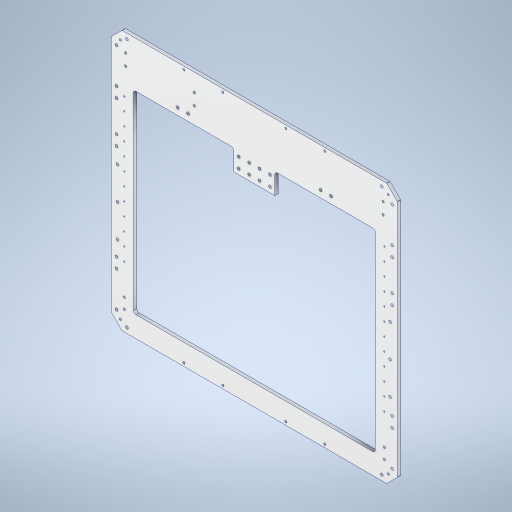
# Autodesk Inventor part: Printer Gantry Plate RevII
Saved by Autodesk Inventor 2024 (Build 280153000, 153)
## iProperties
Created: 2024-10-26
Part Number: Printer Gantry Plate RevII
Material: Aluminum 6061
Document SubType Name: Modeling
Designer: Ishaan
Density: 2.7 g/cm^3
Appearance: Aluminum - Flat
Author: Ishaan
Autodesk Inventor part; units mm, degrees
ref_plane "YZ Plane" through (0, 0, 0) normal (1, 0, 0) x (0, 1, 0)
ref_plane "XZ Plane" through (0, 0, 0) normal (0, 1, 0) x (-1, 0, 0)
ref_plane "XY Plane" through (0, 0, 0) normal (0, 0, 1) x (1, 0, 0)
sketch "Sketch1" plane through (0, 0, 0) normal (0, 0, 1) x (1, 0, 0)
  line L0 (275, -250) -> (-275, -250)
  line L1 (-275, -250) -> (-275, 250)
  line L2 (-275, 250) -> (275, 250)
  line L3 (275, 250) -> (275, -250)
  line L4 (275, -250) -> (-275, 250) construction
  line L5 (-275, -250) -> (275, 250) construction
  point P0 (0, 0)
  dimension "d0" = 550
  dimension "d1" = 500
  constraints: 12 end point, 2 midpoint, 2 parallel, 1 horizontal, 1 perpendicular
  measures "d0" distance of L1.end L2.end
  measures "d1" distance of L0.end L1.end
extrude "Extrusion1" add sketch "Sketch1" against normal blind 6.35
sketch "Sketch2" plane through (0, 0, 0) normal (0, 0, 1) x (1, 0, 0)
  line L0 (-235, 210) -> (-275, 210) construction
  line L1 (-275, 210) -> (-275, 250) construction
  line L2 (-275, 250) -> (-235, 250) construction
  line L3 (-235, 250) -> (-235, 210) construction
  line L4 (-235, 210) -> (-275, 250) construction
  line L5 (-275, 210) -> (-235, 250) construction
  line L6 (275, 210) -> (235, 210) construction
  line L7 (235, 210) -> (235, 250) construction
  line L8 (235, 250) -> (275, 250) construction
  line L9 (275, 250) -> (275, 210) construction
  line L10 (275, 210) -> (235, 250) construction
  line L11 (235, 210) -> (275, 250) construction
  line L12 (40, 122) -> (-40, 122) construction
  line L13 (-40, 122) -> (-40, 162) construction
  line L14 (-40, 162) -> (40, 162) construction
  line L15 (40, 162) -> (40, 122) construction
  line L16 (40, 122) -> (-40, 162) construction
  line L17 (-40, 122) -> (40, 162) construction
  line L18 (-235, -250) -> (-275, -250) construction
  line L19 (-275, -250) -> (-275, -210) construction
  line L20 (-275, -210) -> (-235, -210) construction
  line L21 (-235, -210) -> (-235, -250) construction
  line L22 (-235, -250) -> (-275, -210) construction
  line L23 (-275, -250) -> (-235, -210) construction
  line L24 (-275, 250) -> (-275, -250) construction
  line L25 (-275, -250) -> (275, -250) construction
  line L26 (275, -250) -> (235, -250) construction
  line L27 (235, -250) -> (235, -210) construction
  line L28 (235, -210) -> (275, -210) construction
  line L29 (275, -210) -> (275, -250) construction
  line L30 (275, -250) -> (235, -210) construction
  line L31 (235, -250) -> (275, -210) construction
  line L32 (275, -250) -> (275, 250) construction
  line L33 (-255, 122) -> (-275, 122) construction
  line L34 (-275, 122) -> (-275, 162) construction
  line L35 (-275, 162) -> (-255, 162) construction
  line L36 (-255, 162) -> (-255, 122) construction
  line L37 (-255, 122) -> (-275, 162) construction
  line L38 (-275, 122) -> (-255, 162) construction
  line L39 (275, 122) -> (255, 122) construction
  line L40 (255, 122) -> (255, 162) construction
  line L41 (255, 162) -> (275, 162) construction
  line L42 (275, 162) -> (275, 122) construction
  line L43 (275, 122) -> (255, 162) construction
  line L44 (255, 122) -> (275, 162) construction
  line L45 (-117.5, 165) -> (-157.5, 165) construction
  line L46 (-157.5, 165) -> (-157.5, 185) construction
  line L47 (-157.5, 185) -> (-117.5, 185) construction
  line L48 (-117.5, 185) -> (-117.5, 165) construction
  line L49 (-117.5, 165) -> (-157.5, 185) construction
  line L50 (-157.5, 165) -> (-117.5, 185) construction
  line L51 (157.5, 165) -> (117.5, 165) construction
  line L52 (117.5, 165) -> (117.5, 185) construction
  line L53 (117.5, 185) -> (157.5, 185) construction
  line L54 (157.5, 185) -> (157.5, 165) construction
  line L55 (157.5, 165) -> (117.5, 185) construction
  line L56 (117.5, 165) -> (157.5, 185) construction
  line L57 (-137.5, 175) -> (137.5, 175) construction
  line L58 (-255, -162) -> (-275, -162) construction
  line L59 (-275, -162) -> (-275, -122) construction
  line L60 (-275, -122) -> (-255, -122) construction
  line L61 (-255, -122) -> (-255, -162) construction
  line L62 (-255, -162) -> (-275, -122) construction
  line L63 (-275, -162) -> (-255, -122) construction
  line L64 (-255, 42) -> (-275, 42) construction
  line L65 (-275, 42) -> (-275, 82) construction
  line L66 (-275, 82) -> (-255, 82) construction
  line L67 (-255, 82) -> (-255, 42) construction
  line L68 (-255, 42) -> (-275, 82) construction
  line L69 (-275, 42) -> (-255, 82) construction
  line L70 (275, 42) -> (255, 42) construction
  line L71 (255, 42) -> (255, 82) construction
  line L72 (255, 82) -> (275, 82) construction
  line L73 (275, 82) -> (275, 42) construction
  line L74 (275, 42) -> (255, 82) construction
  line L75 (255, 42) -> (275, 82) construction
  line L76 (275, -162) -> (255, -162) construction
  line L77 (255, -162) -> (255, -122) construction
  line L78 (255, -122) -> (275, -122) construction
  line L79 (275, -122) -> (275, -162) construction
  line L80 (275, -162) -> (255, -122) construction
  line L81 (255, -162) -> (275, -122) construction
  line L82 (-275, 220) -> (-235, 220) construction
  line L83 (-275, -250) -> (-275, 250) construction
  line L84 (-275, 132) -> (-255, 132) construction
  line L85 (-275, -220) -> (-235, -220) construction
  line L86 (-275, -132) -> (-255, -132) construction
  line L87 (-255, 42) -> (-255, -122) construction
  line L88 (-255, -40) -> (0, -40) construction
  line L89 (0, 122) -> (0, -250) construction
  line L90 (-245, 220) -> (-265, 220) construction
  line L91 (-265, 220) -> (-265, 240) construction
  line L92 (-265, 240) -> (-245, 240) construction
  line L93 (-245, 240) -> (-245, 220) construction
  line L94 (-245, 220) -> (-265, 240) construction
  line L95 (-265, 220) -> (-245, 240) construction
  line L96 (265, 220) -> (245, 220) construction
  line L97 (245, 220) -> (245, 240) construction
  line L98 (245, 240) -> (265, 240) construction
  line L99 (265, 240) -> (265, 220) construction
  line L100 (265, 220) -> (245, 240) construction
  line L101 (245, 220) -> (265, 240) construction
  line L102 (265, 152) -> (265, 132) construction
  line L103 (265, 72) -> (265, 52) construction
  line L104 (265, -132) -> (265, -152) construction
  line L105 (-265, 152) -> (-265, 132) construction
  line L106 (-265, 72) -> (-265, 52) construction
  line L107 (-265, -132) -> (-265, -152) construction
  line L108 (-147.5, 175) -> (-127.5, 175) construction
  line L109 (127.5, 175) -> (147.5, 175) construction
  line L110 (265, -240) -> (245, -240) construction
  line L111 (245, -240) -> (245, -220) construction
  line L112 (245, -220) -> (265, -220) construction
  line L113 (265, -220) -> (265, -240) construction
  line L114 (265, -240) -> (245, -220) construction
  line L115 (245, -240) -> (265, -220) construction
  line L116 (-245, -240) -> (-265, -240) construction
  line L117 (-265, -240) -> (-265, -220) construction
  line L118 (-265, -220) -> (-245, -220) construction
  line L119 (-245, -220) -> (-245, -240) construction
  line L120 (-245, -240) -> (-265, -220) construction
  line L121 (-265, -240) -> (-245, -220) construction
  line L122 (10, 132) -> (-10, 132) construction
  line L123 (-10, 132) -> (-10, 152) construction
  line L124 (-10, 152) -> (10, 152) construction
  line L125 (10, 152) -> (10, 132) construction
  line L126 (10, 132) -> (-10, 152) construction
  line L127 (-10, 132) -> (10, 152) construction
  line L128 (30, 132) -> (-30, 132) construction
  line L129 (-30, 132) -> (-30, 152) construction
  line L130 (-30, 152) -> (30, 152) construction
  line L131 (30, 152) -> (30, 132) construction
  line L132 (30, 132) -> (-30, 152) construction
  line L133 (-30, 132) -> (30, 152) construction
  point P0 (0, 0)
  point P1 (-255, 230)
  point P2 (255, 230)
  point P3 (0, 142)
  point P4 (-255, -230)
  point P5 (255, -230)
  point P6 (0, 175)
  point P7 (265, 142)
  point P8 (265, 62)
  point P9 (265, -142)
  point P10 (-265, -142)
  point P11 (-265, 62)
  point P12 (-265, 142)
  point P13 (0, 142)
  dimension "d4" = 40
  dimension "d5" = 40
  dimension "d6" = 40
  dimension "d7" = 40
  dimension "d8" = 80
  dimension "d9" = 40
  dimension "d10" = 40
  dimension "d11" = 40
  dimension "d13" = 40
  dimension "d14" = 40
  dimension "d15" = 20
  dimension "d16" = 40
  dimension "d17" = 20
  dimension "d18" = 40
  dimension "d19" = 40
  dimension "d20" = 20
  dimension "d21" = 40
  dimension "d22" = 20
  dimension "d23" = 3
  dimension "d24" = 275
  dimension "d25" = 20
  dimension "d26" = 40
  dimension "d27" = 20
  dimension "d28" = 40
  dimension "d29" = 20
  dimension "d30" = 40
  dimension "d31" = 20
  dimension "d32" = 40
  dimension "d33" = 392
  dimension "d35" = 10
  dimension "d36" = 10
  dimension "d37" = 88
  dimension "d40" = 88
  dimension "d42" = 48
  dimension "d44" = 164
  dimension "d49" = 10
  dimension "d51" = 162
  dimension "d52" = 20
  dimension "d53" = 20
  dimension "d54" = 20
  dimension "d55" = 20
  dimension "d56" = 20
  dimension "d57" = 20
  dimension "d58" = 20
  dimension "d59" = 20
  dimension "d60" = 20
  dimension "d61" = 20
  dimension "d62" = 20
  dimension "d63" = 20
  dimension "d64" = 20
  dimension "d65" = 20
  dimension "d66" = 20
  dimension "d67" = 20
  dimension "d68" = 20
  dimension "d69" = 20
  dimension "d70" = 60
  dimension "d71" = 20
  dimension "d79" = 10
  dimension "d87" = 80
  constraints: 260 end point, 52 midpoint, 38 parallel, 33 coincident, 23 perpendicular, 22 horizontal, 13 collinear, 6 vertical, 5 point on line, 2 horizontal alignment, 2 vertical alignment, 4 other
  measures "d4" distance of L1.end L2.end
  measures "d5" distance of L0.end L1.end
  measures "d6" distance of L7.end L8.end
  measures "d7" distance of L6.end L7.end
  measures "d8" distance of L13.end L14.end
  measures "d9" distance of L12.end L13.end
  measures "d10" distance of L19.end L20.end
  measures "d11" distance of L18.end L19.end
  measures "d13" distance of L27.end L28.end
  measures "d14" distance of L26.end L27.end
  measures "d15" distance of L34.end L35.end
  measures "d16" distance of L33.end L34.end
  measures "d17" distance of L40.end L41.end
  measures "d18" distance of L39.end L40.end
  measures "d19" distance of L46.end L47.end
  measures "d20" distance of L45.end L46.end
  measures "d21" distance of L52.end L53.end
  measures "d22" distance of L51.end L52.end
  measures "d23" distance between parallel lines of L14 L45
  measures "d24" distance of L57.start L57.end
  measures "d25" distance of L59.end L60.end
  measures "d26" distance of L58.end L59.end
  measures "d27" distance of L65.end L66.end
  measures "d28" distance of L64.end L65.end
  measures "d29" distance of L71.end L72.end
  measures "d30" distance of L70.end L71.end
  measures "d31" distance of L77.end L78.end
  measures "d32" distance of L76.end L77.end
  measures "d33" distance from line of L25 point (0, 142)
  measures "d35" distance between parallel lines of L82 L0
  measures "d36" distance between parallel lines of L33 L84
  measures "d37" distance between parallel lines of L82 L84
  measures "d40" distance between parallel lines of L86 L85
  measures "d42" distance between parallel lines of L20 L58
  measures "d44" distance between parallel lines of L60 L64
  measures "d49" distance between parallel lines of L60 L86
  measures "d51" distance between parallel lines of L12 L88
  measures "d52" distance of L91.end L92.end
  measures "d53" distance of L90.end L91.end
  measures "d54" distance of L97.end L98.end
  measures "d55" distance of L96.end L97.end
  measures "d56" distance of L102.start L102.end
  measures "d57" distance of L103.start L103.end
  measures "d58" distance of L104.start L104.end
  measures "d59" distance of L105.start L105.end
  measures "d60" distance of L106.start L106.end
  measures "d61" distance of L107.start L107.end
  measures "d62" distance of L108.start L108.end
  measures "d63" distance of L109.start L109.end
  measures "d64" distance of L111.end L112.end
  measures "d65" distance of L110.end L111.end
  measures "d66" distance of L117.end L118.end
  measures "d67" distance of L116.end L117.end
  measures "d68" distance of L123.end L124.end
  measures "d69" distance of L122.end L123.end
  measures "d70" distance of L129.end L130.end
  measures "d71" distance of L128.end L129.end
  measures "d79" distance between parallel lines of L20 L85
  measures "d87" distance between parallel lines of L66 L35
hole "Hole1" at (-245, 240, 0) at (-265, 220, 0) at (245, 240, 0) at (265, 220, 0) at (265, 152, 0) at (265, 132, 0) at (265, 52, 0) at (265, 72, 0) at (265, -152, 0) at (265, -132, 0) at (-265, 132, 0) at (-265, 152, 0) at (-265, 52, 0) at (-265, 72, 0) at (-265, -152, 0) at (-265, -132, 0) at (-127.5, 175, 0) at (-147.5, 175, 0) at (147.5, 175, 0) at (127.5, 175, 0) at (-265, -220, 0) at (-245, -240, 0) at (245, -240, 0) at (265, -220, 0) at (-30, 152, 0) at (-30, 132, 0) at (-10, 132, 0) at (-10, 152, 0) at (10, 152, 0) at (10, 132, 0) at (30, 132, 0) at (30, 152, 0) direction (0, 0, -1) diameter 5.3 end through all
sketch "Sketch9" plane through (0, 0, 0) normal (0, 0, 1) x (1, 0, 0)
  line L0 (232.5, -210) -> (-232.5, -210)
  line L1 (-232.5, -210) -> (-232.5, 162)
  line L2 (-232.5, 162) -> (232.5, 162)
  line L3 (232.5, 162) -> (232.5, -210)
  line L4 (232.5, -210) -> (-232.5, 162) construction
  line L5 (-232.5, -210) -> (232.5, 162) construction
  line L6 (-275, -250) -> (275, -250) projected
  circle A0 centre (30, 152) radius 2.65 construction
  circle A1 centre (30, 132) radius 2.65 construction
  circle A2 centre (10, 132) radius 2.65 construction
  circle A3 centre (10, 152) radius 2.65 construction
  circle A4 centre (-10, 152) radius 2.65 construction
  circle A5 centre (-10, 132) radius 2.65 construction
  circle A6 centre (-30, 132) radius 2.65 construction
  circle A7 centre (-30, 152) radius 2.65 construction
  circle A8 centre (265, -220) radius 2.65 construction
  circle A9 centre (245, -240) radius 2.65 construction
  circle A10 centre (-245, -240) radius 2.65 construction
  circle A11 centre (-265, -220) radius 2.65 construction
  circle A12 centre (127.5, 175) radius 2.65 construction
  circle A13 centre (147.5, 175) radius 2.65 construction
  circle A14 centre (-147.5, 175) radius 2.65 construction
  circle A15 centre (-127.5, 175) radius 2.65 construction
  circle A16 centre (-265, -132) radius 2.65 construction
  circle A17 centre (-265, -152) radius 2.65 construction
  circle A18 centre (-265, 72) radius 2.65 construction
  circle A19 centre (-265, 52) radius 2.65 construction
  circle A20 centre (-265, 152) radius 2.65 construction
  circle A21 centre (-265, 132) radius 2.65 construction
  circle A22 centre (265, -132) radius 2.65 construction
  circle A23 centre (265, -152) radius 2.65 construction
  circle A24 centre (265, 72) radius 2.65 construction
  circle A25 centre (265, 52) radius 2.65 construction
  circle A26 centre (265, 132) radius 2.65 construction
  circle A27 centre (265, 152) radius 2.65 construction
  circle A28 centre (265, 220) radius 2.65 construction
  circle A29 centre (245, 240) radius 2.65 construction
  circle A30 centre (-265, 220) radius 2.65 construction
  circle A31 centre (-245, 240) radius 2.65 construction
  line L7 (275, 250) -> (-275, 250) construction
  line L8 (-275, 250) -> (-275, -250) construction
  line L9 (-275, -250) -> (275, -250) construction
  line L10 (275, -250) -> (275, 250) construction
  line L11 (-30, 152) -> (30, 132) construction
  line L12 (39.6, 122) -> (-39.6, 122)
  line L13 (-39.6, 122) -> (-39.6, 162)
  line L14 (-39.6, 162) -> (39.6, 162)
  line L15 (39.6, 162) -> (39.6, 122)
  line L16 (39.6, 122) -> (-39.6, 162) construction
  line L17 (-39.6, 122) -> (39.6, 162) construction
  point P0 (0, 0)
  point P1 (0, -24)
  point P2 (0, 142)
  dimension "d148" = 465
  dimension "d150" = 40
  dimension "d151" = 79.2
  dimension "d152" = 40
  dimension "d153" = 13
  constraints: 26 end point, 5 midpoint, 4 parallel, 2 horizontal, 2 perpendicular, 1 vertical alignment
  measures "d148" distance of L1.end L2.end
  measures "d150" distance between parallel lines of L0 L6
  measures "d151" distance of L13.end L14.end
  measures "d152" distance of L12.end L13.end
  measures "d153" distance from line of L2 A13.centre
extrude "Extrusion4" cut sketch "Sketch9" against normal through all contours L0 L1 L2 L13 L12 L15 L3
sketch "Sketch10" plane through (0, 0, 0) normal (0, 0, 1) x (1, 0, 0)
  line L0 (275, 250) -> (-275, 250) projected
  line L1 (-275, 250) -> (-255, 250)
  line L2 (-255, 250) -> (-255, 230)
  line L3 (-255, 230) -> (-275, 230)
  line L4 (-275, 230) -> (-275, 250)
  line L5 (275, 250) -> (275, -250) projected
  line L6 (275, 250) -> (255, 250)
  line L7 (255, 250) -> (255, 230)
  line L8 (255, 230) -> (275, 230)
  line L9 (275, 230) -> (275, 250)
  line L10 (275, -250) -> (255, -250)
  line L11 (255, -250) -> (255, -230)
  line L12 (255, -230) -> (275, -230)
  line L13 (275, -230) -> (275, -250)
  line L14 (-275, -250) -> (-255, -250)
  line L15 (-255, -250) -> (-255, -230)
  line L16 (-255, -230) -> (-275, -230)
  line L17 (-275, -230) -> (-275, -250)
  point P0 (0, 0)
  point P1 (275, -230)
  point P2 (-255, 250)
  dimension "d156" = 20
  dimension "d157" = 20
  constraints: 32 end point, 8 parallel, 4 horizontal, 4 perpendicular, 3 collinear, 3 equal length, 1 point on line
  measures "d156" distance of L2.end L3.end
  measures "d157" distance of L1.end L2.end
extrude "Extrusion5" cut sketch "Sketch10" against normal through all
sketch "Sketch11" plane through (0, 0, 0) normal (0, 0, 1) x (1, 0, 0)
  line L0 (261, -102.5) -> (-263, -102.5) construction
  line L1 (-263, -102.5) -> (-263, 22.5) construction
  line L2 (-263, 22.5) -> (261, 22.5) construction
  line L3 (261, 22.5) -> (261, -102.5) construction
  line L4 (261, -102.5) -> (-263, 22.5) construction
  line L5 (-263, -102.5) -> (261, 22.5) construction
  circle A0 centre (-265, 52) radius 2.65 construction
  circle A1 centre (265, 52) radius 2.65 construction
  circle A2 centre (-265, -132) radius 2.65 construction
  line L6 (-265, 52) -> (-265, -132) construction
  point P0 (0, 0)
  point P1 (-1, -40)
  point P2 (-265, -40)
  point P3 (-263, -40)
  point P4 (261, -40)
  dimension "d160" = 125
  dimension "d161" = 2
  dimension "d162" = 4
  constraints: 14 end point, 5 midpoint, 4 coincident, 2 parallel, 1 horizontal, 1 horizontal alignment, 1 perpendicular, 1 vertical
  measures "d160" distance of L0.end L1.end
  measures "d161" distance from line of L1 L6.start
  measures "d162" distance from line of A1.centre L3
hole "Hole6" at (-263, 22.5, 0) at (-263, -40, 0) at (-263, -102.5, 0) at (261, 22.5, 0) at (261, -40, 0) at (261, -102.5, 0) direction (0, 0, -1) diameter 5.3 end through all
sketch "Sketch12" plane through (0, 0, 0) normal (0, 0, 1) x (1, 0, 0)
  line L0 (-244, -145) -> (-256, -145) construction
  line L1 (-256, -145) -> (-256, 155) construction
  line L2 (-256, 155) -> (-244, 155) construction
  line L3 (-244, 155) -> (-244, -145) construction
  line L4 (-244, -145) -> (-256, 155) construction
  line L5 (-256, -145) -> (-244, 155) construction
  line L6 (-250, 142.5) -> (-250, -132.5) construction
  line L7 (-275, 230) -> (-275, -230) construction
  line L8 (255, 250) -> (-255, 250) construction
  point P0 (0, 0)
  point P1 (-250, 5)
  point P2 (-250, -107.5)
  point P3 (-250, -82.5)
  point P4 (-250, -57.5)
  point P5 (-250, -32.5)
  point P6 (-250, -7.5)
  point P7 (-250, 17.5)
  point P8 (-250, 42.5)
  point P9 (-250, 67.5)
  point P10 (-250, 92.5)
  point P11 (-250, 117.5)
  point P12 (-250, 142.5)
  dimension "d170" = 12
  dimension "d171" = 300
  dimension "d172" = 275
  dimension "d175" = 25
  dimension "d180" = 25
  dimension "d181" = 95
  constraints: 14 end point, 3 midpoint, 2 parallel, 2 vertical, 1 coincident, 1 horizontal, 1 perpendicular, 11 other
  measures "d170" distance of L1.end L2.end
  measures "d171" distance of L0.end L1.end
  measures "d172" distance of L6.start L6.end
  measures "d175" distance of point (-250, -132.5) point (-250, -107.5)
  measures "d180" distance from line of point (-250, 5) L7
  measures "d181" distance between parallel lines of L8 L2
hole "Hole7" at (-250, -132.5, 0) at (-250, -107.5, 0) at (-250, -82.5, 0) at (-250, -57.5, 0) at (-250, -32.5, 0) at (-250, -7.5, 0) at (-250, 17.5, 0) at (-250, 42.5, 0) at (-250, 67.5, 0) at (-250, 92.5, 0) at (-250, 117.5, 0) at (-250, 142.5, 0) direction (0, 0, -1) diameter 2.459 end through all thread size "M3x0.5" class "6H" standard "ANSI Metric M Profile"
mirror "Mirror1" about plane through (0, 0, 0) normal (1, 0, 0) of "Hole7"
sketch "Sketch13" plane through (0, 0, 0) normal (0, 0, 1) x (1, 0, 0)
  line L0 (247.5, 194) -> (-247.5, 194) construction
  line L1 (-247.5, 194) -> (-247.5, 216) construction
  line L2 (-247.5, 216) -> (247.5, 216) construction
  line L3 (247.5, 216) -> (247.5, 194) construction
  line L4 (247.5, 194) -> (-247.5, 216) construction
  line L5 (-247.5, 194) -> (247.5, 216) construction
  line L6 (-115.5, 194) -> (-115.5, 216) construction
  line L7 (255, 250) -> (-255, 250) construction
  line L8 (-275, 230) -> (-275, -230) construction
  line L9 (250, -212) -> (-250, -212) construction
  line L10 (-250, -212) -> (-250, -192) construction
  line L11 (-250, -192) -> (250, -192) construction
  line L12 (250, -192) -> (250, -212) construction
  line L13 (250, -212) -> (-250, -192) construction
  line L14 (-250, -212) -> (250, -192) construction
  line L15 (-255, -250) -> (255, -250) construction
  point P0 (0, 0)
  point P1 (0, 205)
  point P2 (0, -202)
  dimension "d189" = 22
  dimension "d190" = 34
  dimension "d191" = 27.5
  dimension "d192" = 132
  dimension "d193" = 20
  dimension "d194" = 25
  dimension "d195" = 38
  constraints: 26 end point, 10 coincident, 4 midpoint, 4 parallel, 3 perpendicular, 2 horizontal, 2 point on line, 2 vertical alignment
  measures "d189" distance of L0.end L1.end
  measures "d190" distance between parallel lines of L7 L2
  measures "d191" distance between parallel lines of L8 L1
  measures "d192" distance between parallel lines of L6 L1
  measures "d193" distance of L9.end L10.end
  measures "d194" distance between parallel lines of L10 L8
  measures "d195" distance between parallel lines of L15 L9
hole "Hole8" at (-115.5, 216, 0) at (-115.5, 194, 0) at (-247.5, 216, 0) at (-247.5, 194, 0) at (247.5, 216, 0) at (247.5, 194, 0) at (-250, -192, 0) at (-250, -212, 0) at (250, -192, 0) at (250, -212, 0) direction (0, 0, -1) diameter 4.134 end through all thread size "M5x0.8" class "6H" standard "ANSI Metric M Profile"
fillet "Fillet2" radius 5 4 edges at (-232.5, 162, -3.175) (232.5, 162, -3.175) (232.5, -210, -3.175) (-232.5, -210, -3.175)
fillet "Fillet3" radius 5 2 edges at (-39.6, 162, -3.175) (39.6, 162, -3.175)
fillet "Fillet4" radius 1 12 edges at (255, -250, -3.175) (255, -230, -3.175) (275, -230, -3.175) (255, 230, -3.175) (275, 230, -3.175) (255, 250, -3.175) (-255, -230, -3.175) (-275, 230, -3.175) (-255, 230, -3.175) (-255, 250, -3.175) (-255, -250, -3.175) (-275, -230, -3.175)
sketch "Sketch14" plane through (0, 0, 0) normal (0, 0, 1) x (1, 0, 0)
  circle A0 centre (250, -212) radius 2.067 projected
  circle A1 centre (250, -192) radius 2.067 projected
  circle A2 centre (-250, -212) radius 2.067 projected
  circle A3 centre (-250, -192) radius 2.067 projected
  circle A4 centre (247.5, 194) radius 2.067 projected
  circle A5 centre (247.5, 216) radius 2.067 projected
  circle A6 centre (-247.5, 194) radius 2.067 projected
  circle A7 centre (-247.5, 216) radius 2.067 projected
  circle A8 centre (-115.5, 194) radius 2.067 projected
  circle A9 centre (-115.5, 216) radius 2.067 projected
  circle A10 centre (250, 142.5) radius 1.2295 projected
  circle A11 centre (250, -132.5) radius 1.2295 projected
  circle A12 centre (250, -107.5) radius 1.2295 projected
  circle A13 centre (250, -82.5) radius 1.2295 projected
  circle A14 centre (250, -57.5) radius 1.2295 projected
  circle A15 centre (250, -32.5) radius 1.2295 projected
  circle A16 centre (250, -7.5) radius 1.2295 projected
  circle A17 centre (250, 17.5) radius 1.2295 projected
  circle A18 centre (250, 42.5) radius 1.2295 projected
  circle A19 centre (250, 67.5) radius 1.2295 projected
  circle A20 centre (250, 92.5) radius 1.2295 projected
  circle A21 centre (250, 117.5) radius 1.2295 projected
  circle A22 centre (-250, 142.5) radius 1.2295 projected
  circle A23 centre (-250, 117.5) radius 1.2295 projected
  circle A24 centre (-250, 92.5) radius 1.2295 projected
  circle A25 centre (-250, 67.5) radius 1.2295 projected
  circle A26 centre (-250, 42.5) radius 1.2295 projected
  circle A27 centre (-250, 17.5) radius 1.2295 projected
  circle A28 centre (-250, -7.5) radius 1.2295 projected
  circle A29 centre (-250, -32.5) radius 1.2295 projected
  circle A30 centre (-250, -57.5) radius 1.2295 projected
  circle A31 centre (-250, -82.5) radius 1.2295 projected
  circle A32 centre (-250, -107.5) radius 1.2295 projected
  circle A33 centre (-250, -132.5) radius 1.2295 projected
  circle A34 centre (261, -102.5) radius 2.65 projected
  circle A35 centre (261, -40) radius 2.65 projected
  circle A36 centre (261, 22.5) radius 2.65 projected
  circle A37 centre (-263, -102.5) radius 2.65 projected
  circle A38 centre (-263, -40) radius 2.65 projected
  circle A39 centre (-263, 22.5) radius 2.65 projected
  arc A40 (-275, -229) -> (-274, -230) centre (-274, -229) ccw projected
  line L0 (-274, -230) -> (-256, -230) projected
  arc A41 (-255, -231) -> (-256, -230) centre (-256, -231) ccw projected
  line L1 (-255, -231) -> (-255, -249) projected
  arc A42 (-255, -249) -> (-254, -250) centre (-254, -249) ccw projected
  line L2 (-254, -250) -> (254, -250) projected
  arc A43 (254, -250) -> (255, -249) centre (254, -249) ccw projected
  line L3 (255, -249) -> (255, -231) projected
  arc A44 (256, -230) -> (255, -231) centre (256, -231) ccw projected
  line L4 (256, -230) -> (274, -230) projected
  arc A45 (274, -230) -> (275, -229) centre (274, -229) ccw projected
  line L5 (275, -229) -> (275, 229) projected
  arc A46 (275, 229) -> (274, 230) centre (274, 229) ccw projected
  line L6 (274, 230) -> (256, 230) projected
  arc A47 (255, 231) -> (256, 230) centre (256, 231) ccw projected
  line L7 (255, 231) -> (255, 249) projected
  arc A48 (255, 249) -> (254, 250) centre (254, 249) ccw projected
  line L8 (254, 250) -> (-254, 250) projected
  arc A49 (-254, 250) -> (-255, 249) centre (-254, 249) ccw projected
  line L9 (-255, 249) -> (-255, 231) projected
  arc A50 (-256, 230) -> (-255, 231) centre (-256, 231) ccw projected
  line L10 (-256, 230) -> (-274, 230) projected
  arc A51 (-274, 230) -> (-275, 229) centre (-274, 229) ccw projected
  line L11 (-275, 229) -> (-275, -229) projected
  line L12 (232.5, 157) -> (232.5, -205) projected
  arc A52 (227.5, -210) -> (232.5, -205) centre (227.5, -205) ccw projected
  line L13 (227.5, -210) -> (-227.5, -210) projected
  arc A53 (-232.5, -205) -> (-227.5, -210) centre (-227.5, -205) ccw projected
  line L14 (-232.5, -205) -> (-232.5, 157) projected
  arc A54 (-227.5, 162) -> (-232.5, 157) centre (-227.5, 157) ccw projected
  line L15 (-227.5, 162) -> (-44.6, 162) projected
  arc A55 (-39.6, 157) -> (-44.6, 162) centre (-44.6, 157) ccw projected
  line L16 (-39.6, 157) -> (-39.6, 122) projected
  line L17 (-39.6, 122) -> (39.6, 122) projected
  line L18 (39.6, 122) -> (39.6, 157) projected
  arc A56 (44.6, 162) -> (39.6, 157) centre (44.6, 157) ccw projected
  line L19 (44.6, 162) -> (227.5, 162) projected
  arc A57 (232.5, 157) -> (227.5, 162) centre (227.5, 157) ccw projected
  circle A58 centre (30, 152) radius 2.65 projected
  circle A59 centre (30, 132) radius 2.65 projected
  circle A60 centre (10, 132) radius 2.65 projected
  circle A61 centre (10, 152) radius 2.65 projected
  circle A62 centre (-10, 152) radius 2.65 projected
  circle A63 centre (-10, 132) radius 2.65 projected
  circle A64 centre (-30, 132) radius 2.65 projected
  circle A65 centre (-30, 152) radius 2.65 projected
  circle A66 centre (265, -220) radius 2.65 projected
  circle A67 centre (245, -240) radius 2.65 projected
  circle A68 centre (-245, -240) radius 2.65 projected
  circle A69 centre (-265, -220) radius 2.65 projected
  circle A70 centre (127.5, 175) radius 2.65 projected
  circle A71 centre (147.5, 175) radius 2.65 projected
  circle A72 centre (-147.5, 175) radius 2.65 projected
  circle A73 centre (-127.5, 175) radius 2.65 projected
  circle A74 centre (-265, -132) radius 2.65 projected
  circle A75 centre (-265, -152) radius 2.65 projected
  circle A76 centre (-265, 72) radius 2.65 projected
  circle A77 centre (-265, 52) radius 2.65 projected
  circle A78 centre (-265, 152) radius 2.65 projected
  circle A79 centre (-265, 132) radius 2.65 projected
  circle A80 centre (265, -132) radius 2.65 projected
  circle A81 centre (265, -152) radius 2.65 projected
  circle A82 centre (265, 72) radius 2.65 projected
  circle A83 centre (265, 52) radius 2.65 projected
  circle A84 centre (265, 132) radius 2.65 projected
  circle A85 centre (265, 152) radius 2.65 projected
  circle A86 centre (265, 220) radius 2.65 projected
  circle A87 centre (245, 240) radius 2.65 projected
  circle A88 centre (-265, 220) radius 2.65 projected
  circle A89 centre (-245, 240) radius 2.65 projected
  arc A90 (255, 249) -> (254, 250) centre (254, 249) ccw projected
  line L20 (0, 504.4142) -> (504.4142, 0)
  line L21 (504.4142, 0) -> (0, -504.4142)
  line L22 (0, -504.4142) -> (-504.4142, 0)
  line L23 (-504.4142, 0) -> (0, 504.4142)
  arc A91 (274, -230) -> (275, -229) centre (274, -229) ccw projected
  point P0 (0, 0)
  point P1 (254.7071, -249.7071)
  point P2 (274.7071, -229.7071)
  point P3 (274.7071, 229.7071)
  point P4 (254.7071, 249.7071)
  point P5 (-254.7071, 249.7071)
  point P6 (-274.7071, 229.7071)
  point P7 (-274.7071, -229.7071)
  point P8 (-254.7071, -249.7071)
  constraints: 8 end point, 5 tangent, 2 parallel, 1 perpendicular
extrude "Extrusion6" add sketch "Sketch14" against normal up to surface (6.35 mm away) contours A40 L0 A41 L1 A42 L22 | L23 A49 L9 A50 L10 A51 | A43 L3 A44 L4 A45 L21 | L20 A46 L6 A47 L7 A48
sketch "Sketch15" plane through (0, 0, 0) normal (0, 0, 1) x (1, 0, 0)
  circle A0 centre (250, -212) radius 2.067 projected
  circle A1 centre (250, -192) radius 2.067 projected
  circle A2 centre (-250, -212) radius 2.067 projected
  circle A3 centre (-250, -192) radius 2.067 projected
  circle A4 centre (247.5, 194) radius 2.067 projected
  circle A5 centre (247.5, 216) radius 2.067 projected
  circle A6 centre (-247.5, 194) radius 2.067 projected
  circle A7 centre (-247.5, 216) radius 2.067 projected
  circle A8 centre (-115.5, 194) radius 2.067 projected
  circle A9 centre (-115.5, 216) radius 2.067 projected
  circle A10 centre (250, 142.5) radius 1.2295 projected
  circle A11 centre (250, -132.5) radius 1.2295 projected
  circle A12 centre (250, -107.5) radius 1.2295 projected
  circle A13 centre (250, -82.5) radius 1.2295 projected
  circle A14 centre (250, -57.5) radius 1.2295 projected
  circle A15 centre (250, -32.5) radius 1.2295 projected
  circle A16 centre (250, -7.5) radius 1.2295 projected
  circle A17 centre (250, 17.5) radius 1.2295 projected
  circle A18 centre (250, 42.5) radius 1.2295 projected
  circle A19 centre (250, 67.5) radius 1.2295 projected
  circle A20 centre (250, 92.5) radius 1.2295 projected
  circle A21 centre (250, 117.5) radius 1.2295 projected
  circle A22 centre (-250, 142.5) radius 1.2295 projected
  circle A23 centre (-250, 117.5) radius 1.2295 projected
  circle A24 centre (-250, 92.5) radius 1.2295 projected
  circle A25 centre (-250, 67.5) radius 1.2295 projected
  circle A26 centre (-250, 42.5) radius 1.2295 projected
  circle A27 centre (-250, 17.5) radius 1.2295 projected
  circle A28 centre (-250, -7.5) radius 1.2295 projected
  circle A29 centre (-250, -32.5) radius 1.2295 projected
  circle A30 centre (-250, -57.5) radius 1.2295 projected
  circle A31 centre (-250, -82.5) radius 1.2295 projected
  circle A32 centre (-250, -107.5) radius 1.2295 projected
  circle A33 centre (-250, -132.5) radius 1.2295 projected
  circle A34 centre (261, -102.5) radius 2.65 projected
  circle A35 centre (261, -40) radius 2.65 projected
  circle A36 centre (261, 22.5) radius 2.65 projected
  circle A37 centre (-263, -102.5) radius 2.65 projected
  circle A38 centre (-263, -40) radius 2.65 projected
  circle A39 centre (-263, 22.5) radius 2.65 projected
  line L0 (-274.7071, -229.7071) -> (-254.7071, -249.7071) projected
  arc A40 (-254.7071, -249.7071) -> (-254, -250) centre (-254, -249) ccw projected
  line L1 (-254, -250) -> (254, -250) projected
  arc A41 (254, -250) -> (254.7071, -249.7071) centre (254, -249) ccw projected
  line L2 (254.7071, -249.7071) -> (274.7071, -229.7071) projected
  arc A42 (274.7071, -229.7071) -> (275, -229) centre (274, -229) ccw projected
  line L3 (275, -229) -> (275, 229) projected
  arc A43 (275, 229) -> (274.7071, 229.7071) centre (274, 229) ccw projected
  line L4 (274.7071, 229.7071) -> (254.7071, 249.7071) projected
  arc A44 (254.7071, 249.7071) -> (254, 250) centre (254, 249) ccw projected
  line L5 (254, 250) -> (-254, 250) projected
  arc A45 (-254, 250) -> (-254.7071, 249.7071) centre (-254, 249) ccw projected
  line L6 (-254.7071, 249.7071) -> (-274.7071, 229.7071) projected
  arc A46 (-274.7071, 229.7071) -> (-275, 229) centre (-274, 229) ccw projected
  line L7 (-275, 229) -> (-275, -229) projected
  arc A47 (-275, -229) -> (-274.7071, -229.7071) centre (-274, -229) ccw projected
  line L8 (232.5, 157) -> (232.5, -205) projected
  arc A48 (227.5, -210) -> (232.5, -205) centre (227.5, -205) ccw projected
  line L9 (227.5, -210) -> (-227.5, -210) projected
  arc A49 (-232.5, -205) -> (-227.5, -210) centre (-227.5, -205) ccw projected
  line L10 (-232.5, -205) -> (-232.5, 157) projected
  arc A50 (-227.5, 162) -> (-232.5, 157) centre (-227.5, 157) ccw projected
  line L11 (-227.5, 162) -> (-44.6, 162) projected
  arc A51 (-39.6, 157) -> (-44.6, 162) centre (-44.6, 157) ccw projected
  line L12 (-39.6, 157) -> (-39.6, 122) projected
  line L13 (-39.6, 122) -> (39.6, 122) projected
  line L14 (39.6, 122) -> (39.6, 157) projected
  arc A52 (44.6, 162) -> (39.6, 157) centre (44.6, 157) ccw projected
  line L15 (44.6, 162) -> (227.5, 162) projected
  arc A53 (232.5, 157) -> (227.5, 162) centre (227.5, 157) ccw projected
  circle A54 centre (30, 152) radius 2.65 projected
  circle A55 centre (30, 132) radius 2.65 projected
  circle A56 centre (10, 132) radius 2.65 projected
  circle A57 centre (10, 152) radius 2.65 projected
  circle A58 centre (-10, 152) radius 2.65 projected
  circle A59 centre (-10, 132) radius 2.65 projected
  circle A60 centre (-30, 132) radius 2.65 projected
  circle A61 centre (-30, 152) radius 2.65 projected
  circle A62 centre (265, -220) radius 2.65 projected
  circle A63 centre (245, -240) radius 2.65 projected
  circle A64 centre (-245, -240) radius 2.65 projected
  circle A65 centre (-265, -220) radius 2.65 projected
  circle A66 centre (127.5, 175) radius 2.65 projected
  circle A67 centre (147.5, 175) radius 2.65 projected
  circle A68 centre (-147.5, 175) radius 2.65 projected
  circle A69 centre (-127.5, 175) radius 2.65 projected
  circle A70 centre (-265, -132) radius 2.65 projected
  circle A71 centre (-265, -152) radius 2.65 projected
  circle A72 centre (-265, 72) radius 2.65 projected
  circle A73 centre (-265, 52) radius 2.65 projected
  circle A74 centre (-265, 152) radius 2.65 projected
  circle A75 centre (-265, 132) radius 2.65 projected
  circle A76 centre (265, -132) radius 2.65 projected
  circle A77 centre (265, -152) radius 2.65 projected
  circle A78 centre (265, 72) radius 2.65 projected
  circle A79 centre (265, 52) radius 2.65 projected
  circle A80 centre (265, 132) radius 2.65 projected
  circle A81 centre (265, 152) radius 2.65 projected
  circle A82 centre (265, 220) radius 2.65 projected
  circle A83 centre (245, 240) radius 2.65 projected
  circle A84 centre (-265, 220) radius 2.65 projected
  circle A85 centre (-245, 240) radius 2.65 projected
  line L16 (-257.5, 232.5) -> (257.5, 232.5)
  line L17 (257.5, 232.5) -> (257.5, -232.5)
  line L18 (257.5, -232.5) -> (-257.5, -232.5)
  line L19 (-257.5, -232.5) -> (-257.5, 232.5)
  point P0 (0, 0)
  dimension "d208" = 17.5
  dimension "d209" = 17.5
  dimension "d210" = 17.5
  dimension "d211" = 17.5
  constraints: 8 end point, 4 coincident, 2 parallel, 1 horizontal, 1 perpendicular
  measures "d208" distance between parallel lines of L18 L1
  measures "d209" distance between parallel lines of L3 L17
  measures "d210" distance between parallel lines of L5 L16
  measures "d211" distance between parallel lines of L19 L7
hole "Hole9" at (-257.5, 232.5, 0) at (257.5, 232.5, 0) at (257.5, -232.5, 0) at (-257.5, -232.5, 0) direction (0, 0, -1) diameter 4.134 end through all thread size "M5x0.8" class "6H" standard "ANSI Metric M Profile"
sketch "Sketch16" plane through (0, 0, 0) normal (0, 0, 1) x (1, 0, 0)
  circle A0 centre (-257.5, -232.5) radius 2.067 projected
  circle A1 centre (257.5, -232.5) radius 2.067 projected
  circle A2 centre (257.5, 232.5) radius 2.067 projected
  circle A3 centre (-257.5, 232.5) radius 2.067 projected
  circle A4 centre (250, -212) radius 2.067 projected
  circle A5 centre (250, -192) radius 2.067 projected
  circle A6 centre (-250, -212) radius 2.067 projected
  circle A7 centre (-250, -192) radius 2.067 projected
  circle A8 centre (247.5, 194) radius 2.067 projected
  circle A9 centre (247.5, 216) radius 2.067 projected
  circle A10 centre (-247.5, 194) radius 2.067 projected
  circle A11 centre (-247.5, 216) radius 2.067 projected
  circle A12 centre (-115.5, 194) radius 2.067 projected
  circle A13 centre (-115.5, 216) radius 2.067 projected
  circle A14 centre (250, 142.5) radius 1.2295 projected
  circle A15 centre (250, -132.5) radius 1.2295 projected
  circle A16 centre (250, -107.5) radius 1.2295 projected
  circle A17 centre (250, -82.5) radius 1.2295 projected
  circle A18 centre (250, -57.5) radius 1.2295 projected
  circle A19 centre (250, -32.5) radius 1.2295 projected
  circle A20 centre (250, -7.5) radius 1.2295 projected
  circle A21 centre (250, 17.5) radius 1.2295 projected
  circle A22 centre (250, 42.5) radius 1.2295 projected
  circle A23 centre (250, 67.5) radius 1.2295 projected
  circle A24 centre (250, 92.5) radius 1.2295 projected
  circle A25 centre (250, 117.5) radius 1.2295 projected
  circle A26 centre (-250, 142.5) radius 1.2295 projected
  circle A27 centre (-250, 117.5) radius 1.2295 projected
  circle A28 centre (-250, 92.5) radius 1.2295 projected
  circle A29 centre (-250, 67.5) radius 1.2295 projected
  circle A30 centre (-250, 42.5) radius 1.2295 projected
  circle A31 centre (-250, 17.5) radius 1.2295 projected
  circle A32 centre (-250, -7.5) radius 1.2295 projected
  circle A33 centre (-250, -32.5) radius 1.2295 projected
  circle A34 centre (-250, -57.5) radius 1.2295 projected
  circle A35 centre (-250, -82.5) radius 1.2295 projected
  circle A36 centre (-250, -107.5) radius 1.2295 projected
  circle A37 centre (-250, -132.5) radius 1.2295 projected
  circle A38 centre (261, -102.5) radius 2.65 projected
  circle A39 centre (261, -40) radius 2.65 projected
  circle A40 centre (261, 22.5) radius 2.65 projected
  circle A41 centre (-263, -102.5) radius 2.65 projected
  circle A42 centre (-263, -40) radius 2.65 projected
  circle A43 centre (-263, 22.5) radius 2.65 projected
  line L0 (-274.7071, -229.7071) -> (-254.7071, -249.7071) projected
  arc A44 (-254.7071, -249.7071) -> (-254, -250) centre (-254, -249) ccw projected
  line L1 (-254, -250) -> (254, -250) projected
  arc A45 (254, -250) -> (254.7071, -249.7071) centre (254, -249) ccw projected
  line L2 (254.7071, -249.7071) -> (274.7071, -229.7071) projected
  arc A46 (274.7071, -229.7071) -> (275, -229) centre (274, -229) ccw projected
  line L3 (275, -229) -> (275, 229) projected
  arc A47 (275, 229) -> (274.7071, 229.7071) centre (274, 229) ccw projected
  line L4 (274.7071, 229.7071) -> (254.7071, 249.7071) projected
  arc A48 (254.7071, 249.7071) -> (254, 250) centre (254, 249) ccw projected
  line L5 (254, 250) -> (-254, 250) projected
  arc A49 (-254, 250) -> (-254.7071, 249.7071) centre (-254, 249) ccw projected
  line L6 (-254.7071, 249.7071) -> (-274.7071, 229.7071) projected
  arc A50 (-274.7071, 229.7071) -> (-275, 229) centre (-274, 229) ccw projected
  line L7 (-275, 229) -> (-275, -229) projected
  arc A51 (-275, -229) -> (-274.7071, -229.7071) centre (-274, -229) ccw projected
  line L8 (232.5, 157) -> (232.5, -205) projected
  arc A52 (227.5, -210) -> (232.5, -205) centre (227.5, -205) ccw projected
  line L9 (227.5, -210) -> (-227.5, -210) projected
  arc A53 (-232.5, -205) -> (-227.5, -210) centre (-227.5, -205) ccw projected
  line L10 (-232.5, -205) -> (-232.5, 157) projected
  arc A54 (-227.5, 162) -> (-232.5, 157) centre (-227.5, 157) ccw projected
  line L11 (-227.5, 162) -> (-44.6, 162) projected
  arc A55 (-39.6, 157) -> (-44.6, 162) centre (-44.6, 157) ccw projected
  line L12 (-39.6, 157) -> (-39.6, 122) projected
  line L13 (-39.6, 122) -> (39.6, 122) projected
  line L14 (39.6, 122) -> (39.6, 157) projected
  arc A56 (44.6, 162) -> (39.6, 157) centre (44.6, 157) ccw projected
  line L15 (44.6, 162) -> (227.5, 162) projected
  arc A57 (232.5, 157) -> (227.5, 162) centre (227.5, 157) ccw projected
  circle A58 centre (30, 152) radius 2.65 projected
  circle A59 centre (30, 132) radius 2.65 projected
  circle A60 centre (10, 132) radius 2.65 projected
  circle A61 centre (10, 152) radius 2.65 projected
  circle A62 centre (-10, 152) radius 2.65 projected
  circle A63 centre (-10, 132) radius 2.65 projected
  circle A64 centre (-30, 132) radius 2.65 projected
  circle A65 centre (-30, 152) radius 2.65 projected
  circle A66 centre (265, -220) radius 2.65 projected
  circle A67 centre (245, -240) radius 2.65 projected
  circle A68 centre (-245, -240) radius 2.65 projected
  circle A69 centre (-265, -220) radius 2.65 projected
  circle A70 centre (127.5, 175) radius 2.65 projected
  circle A71 centre (147.5, 175) radius 2.65 projected
  circle A72 centre (-147.5, 175) radius 2.65 projected
  circle A73 centre (-127.5, 175) radius 2.65 projected
  circle A74 centre (-265, -132) radius 2.65 projected
  circle A75 centre (-265, -152) radius 2.65 projected
  circle A76 centre (-265, 72) radius 2.65 projected
  circle A77 centre (-265, 52) radius 2.65 projected
  circle A78 centre (-265, 152) radius 2.65 projected
  circle A79 centre (-265, 132) radius 2.65 projected
  circle A80 centre (265, -132) radius 2.65 projected
  circle A81 centre (265, -152) radius 2.65 projected
  circle A82 centre (265, 72) radius 2.65 projected
  circle A83 centre (265, 52) radius 2.65 projected
  circle A84 centre (265, 132) radius 2.65 projected
  circle A85 centre (265, 152) radius 2.65 projected
  circle A86 centre (265, 220) radius 2.65 projected
  circle A87 centre (245, 240) radius 2.65 projected
  circle A88 centre (-265, 220) radius 2.65 projected
  circle A89 centre (-245, 240) radius 2.65 projected
  line L16 (-135.5, -244) -> (-60.5, -244)
  line L17 (60.5, -244) -> (135.5, -244)
  line L18 (-254, -250) -> (254, -250) construction
  line L19 (-98, -244) -> (98, -244) construction
  point P0 (0, 0)
  point P1 (0, -244)
  point P2 (0, -244)
  dimension "d227" = 75
  dimension "d228" = 75
  dimension "d229" = 6
  dimension "d230" = 196
  constraints: 6 end point, 5 coincident, 3 midpoint, 2 horizontal, 1 collinear, 1 vertical alignment
  measures "d227" distance of L16.start L16.end
  measures "d228" distance of L17.start L17.end
  measures "d229" distance between parallel lines of L16 L18
  measures "d230" distance of L19.start L19.end
hole "Hole10" at (-135.5, -244, 0) at (-60.5, -244, 0) at (60.5, -244, 0) at (135.5, -244, 0) direction (0, 0, -1) diameter 4.134 end through all thread size "M5x0.8" class "6H" standard "ANSI Metric M Profile"
mirror "Mirror2" about plane through (0, 0, 0) normal (0, 1, 0) of "Hole10"
equation "\"d40\" = d37"
body "Solid1"
